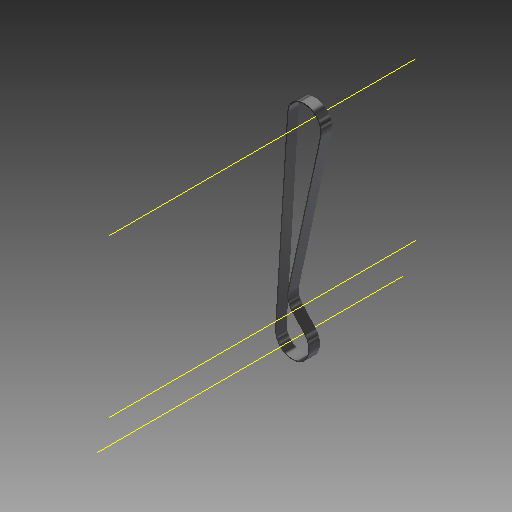
# Autodesk Inventor part: Synchronous Belt
Saved by Autodesk Inventor 2019.4 (Build 234330000, 330)
## iProperties
Created: 2020-01-23
Part Number: Synchronous Belt
Material: Rubber
Document SubType Name: Modeling
Designer: admin
Density: 0.93 g/cm^3
Appearance: Rubber - Black - Version 1.1
Mass: 3.4875 g
Surface Area: 82.5 cm^2
Volume: 3.75 cm^3
CustomPartVersion: 1
Author: admin
Autodesk Inventor part; units mm, degrees
ref_plane "YZ Plane" through (0, 0, 0) normal (1, 0, 0) x (0, 1, 0)
ref_plane "XZ Plane" through (0, 0, 0) normal (0, 1, 0) x (-1, 0, 0)
ref_plane "XY Plane" through (0, 0, 0) normal (0, 0, 1) x (1, 0, 0)
sketch "Sketch Path" plane through (0, 0, 0) normal (0, 0, 1) x (1, 0, 0)
  arc A0 (40.149, -119.2706) -> (67.8241, -109.5644) centre (56.034, -120.2553) ccw
  arc A1 (83.0398, 61.1235) -> (51.6018, 65.4856) centre (67.4868, 64.5009) ccw
  arc A2 (51.9338, -82.1217) -> (55.6967, -96.19) centre (67.4868, -85.4991) ccw
  line L0 (55.6967, -96.19) -> (67.8241, -109.5644)
  line L1 (40.149, -119.2706) -> (51.6018, 65.4856)
  line L2 (83.0398, 61.1235) -> (51.9338, -82.1217)
  constraints: 6 end point, 6 point on circle, 3 centre point
ref_plane "Cross Section Plane" through (67.8241, -109.5644, 0) normal (-0.6717317, 0.7407945, 0) x (0, 0, 1)
ref_plane "Work Plane2" through (56.034, -120.2553, 0) normal (-1, 0, 0) x (0, 0, 1)
ref_plane "Work Plane3" through (67.4868, 64.5009, 0) normal (-0.3023865, -0.9531854, 0) x (0, 0, 1)
ref_plane "Work Plane4" through (67.4868, -85.4991, 0) normal (-0.0628567, -0.9980226, 0) x (0, 0, 1)
sketch "Cross Section" plane through (67.8241, -109.5644, 0) normal (-0.6717317, 0.7407945, 0) x (0, 0, 1)
  line L0 (-5, 0.5) -> (5, 0.5)
  line L1 (5, 0.5) -> (5, -0.5)
  line L2 (5, -0.5) -> (-5, -0.5)
  line L3 (-5, -0.5) -> (-5, 0.5)
  line L4 (-5, 0) -> (5, 0) construction
  point P0 (0, 0)
  point P1 (0, 0)
  dimension "d0" = 10
  dimension "d4" = 0.5
  dimension "d5" = 0.5
  constraints: 10 end point, 3 midpoint, 2 parallel, 1 coincident, 1 horizontal, 1 perpendicular, 1 other
  measures "d0" distance between parallel lines of L1 L3
  measures "d4" distance between parallel lines of L2 L4
  measures "d5" distance between parallel lines of L4 L0
sweep "Belt" add profiles "Cross Section" path "Sketch Path" path curves L2 A2 L0 A0 L1 A1
equation "\"d0\" = da_B"
equation "\"d4\" = da_a"
equation "\"d5\" = da_a2"
equation "\"da_B\" = 10"
equation "\"da_pb\" = 5"
equation "\"da_a\" = 0.5"
equation "\"da_S\" = 2.65"
equation "\"da_Beta\" = 20deg"
equation "\"da_Ht\" = 1.2"
equation "\"da_H\" = 3.4"
equation "\"da_a2\" = 0.5"
body "Solid1"
